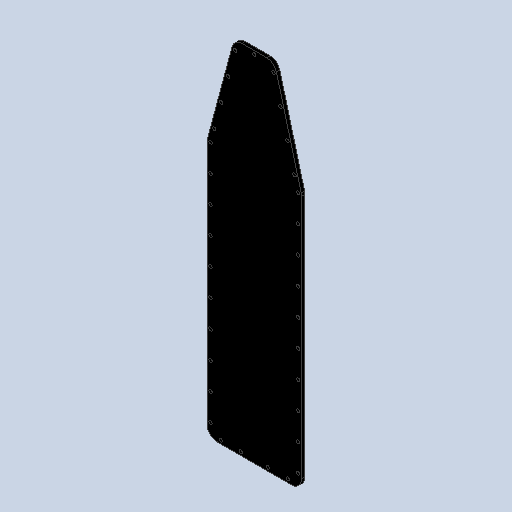
# Autodesk Inventor part: Model Shell - access panel L
Saved by Autodesk Inventor 2023 (Build 270158000, 158)
## iProperties
Created: 2022-12-13
Part Number: Model Shell - access panel L
Material: ABS Plastic
Document SubType Name: Modeling
Designer: Tanzu
Density: 1.06 g/cm^3
Appearance: Aluminum - Polished
Mass: 375.26 g
Surface Area: 1823.85 cm^2
Volume: 354.019 cm^3
Author: Tanzu
Autodesk Inventor part; units mm, degrees
ref_plane "YZ Plane" through (0, 0, 0) normal (1, 0, 0) x (0, 1, 0)
ref_plane "XZ Plane" through (0, 0, 0) normal (0, 1, 0) x (-1, 0, 0)
ref_plane "XY Plane" through (0, 0, 0) normal (0, 0, 1) x (1, 0, 0)
sketch "Sketch2" plane through (0, 0, 0) normal (0, 0, 1) x (1, 0, 0)
  line L0 (-90, 0) -> (90, 0) construction
  line L1 (90, 0) -> (90, 900) construction
  line L2 (90, 900) -> (-90, 900) construction
  line L3 (-90, 900) -> (-90, 0) construction
  line L4 (-90, 250) -> (90, 250) construction
  line L5 (0, 900) -> (90, 564.1154)
  line L6 (0, 900) -> (-90, 564.1154)
  line L7 (0, 900) -> (0, 250) construction
  line L8 (-132.5, 0) -> (132.5, 0) construction
  line L9 (-90, 564.1154) -> (-90, 0)
  line L10 (90, 564.1154) -> (90, 0)
  line L11 (90, 0) -> (-90, 0)
  line L12 (-85, 563.4572) -> (0, 880.6815)
  line L13 (0, 880.6815) -> (85, 563.4572)
  line L14 (85, 563.4572) -> (85, 5)
  line L15 (85, 5) -> (-85, 5)
  line L16 (-85, 5) -> (-85, 563.4572)
  point P0 (0, 0)
  point P1 (0, 0)
  dimension "d4" = 180
  dimension "d5" = 900
  dimension "d6" = 250
  dimension "d7" = 15
  dimension "d8" = 15
  dimension "d9" = 265
  dimension "d10" = 5
  constraints: 34 end point, 4 midpoint, 4 point on line, 3 collinear, 2 horizontal, 2 parallel, 2 perpendicular, 1 coincident, 4 other
  measures "d4" distance of L0.start L0.end
  measures "d5" distance of L0.end L1.end
  measures "d6" distance between parallel lines of L0 L4
  measures "d7" angle of L7 L5
  measures "d8" angle of L6 L7
  measures "d9" distance of L8.start L8.end
  measures "d10" distance between parallel lines of L6 L12
extrude "Extrusion2" add sketch "Sketch2" along normal mid plane 180 contours L5 L10 L11 L9 L6 | L12 L13 L14 L15 L16
sketch "Sketch3" plane through (0, 0, 0) normal (0, 0, 1) x (1, 0, 0)
  line L0 (-132.5, 0) -> (132.5, 0)
  line L1 (-90, 0) -> (90, 0) projected
  line L2 (0, 0) -> (0, 600)
  line L3 (0, 600) -> (-132.5, 0)
  line L4 (0, 601.0824) -> (0, 600)
  line L5 (0, 577.3585) -> (-127.5, 0)
  line L6 (0, 577.3585) -> (0, 601.0824)
  point P0 (0, 0)
  dimension "d13" = 265
  dimension "d14" = 600
  dimension "d17" = 5
  constraints: 12 end point, 3 point on line, 2 midpoint, 2 vertical, 1 collinear, 1 horizontal, 1 parallel
  measures "d13" distance of L0.start L0.end
  measures "d14" distance of L2.start L2.end
  measures "d17" distance of L0.start L5.end
revolve "Revolution1" add sketch "Sketch3" angle 360 about axis through (0, 0, 0) along (0, 1, 0)
revolve "Revolution2" cut sketch "Sketch3" angle 360 about axis through (0, 0, 0) along (0, 1, 0) contours L5 L2 L0
extrude "Extrusion3" cut sketch "Sketch2" along normal mid plane 170 contours L12 L13 L14 L15 L16
sketch "Sketch5" plane through (0, 0, 0) normal (0, -1, 0) x (1, 0, 0)
  circle A0 centre (0, 0) radius 127.5 projected
  circle A1 centre (0, 0) radius 132.5 projected
extrude "Extrusion4" add sketch "Sketch5" along normal blind 100
fillet "Fillet1" radius 10 5 edges at (0, 192.4528, -90) (90, 192.4528, 0) (0, 192.4528, 90) (-90, 152.2344, -40.9581) (-90, 152.2344, 40.9581)
fillet "Fillet2" radius 30 2 edges at (0, 0, 132.5) (0, 0, -132.5)
sketch "Sketch6" plane through (90, 564.1154, 90) normal (1, 0, 0) x (0, 0, -1)
  line L0 (180, 0) -> (180, -526.9621) projected
  line L1 (180, 0) -> (0, 0) projected
  line L2 (0, -526.9621) -> (0, 0) projected
  line L3 (27.5, -275) -> (152.5, -275)
  line L4 (152.5, -275) -> (152.5, -75)
  line L5 (152.5, -75) -> (27.5, -75)
  line L6 (27.5, -75) -> (27.5, -275)
  point P0 (90, -564.1154)
  point P1 (90, 0)
  point P2 (90, -75)
  dimension "d25" = 75
  dimension "d26" = 200
  dimension "d27" = 125
  constraints: 8 end point, 2 midpoint, 2 parallel, 1 horizontal, 1 horizontal alignment, 1 perpendicular, 1 vertical alignment
  measures "d25" distance between parallel lines of L1 L5
  measures "d26" distance of L5.end L3.start
  measures "d27" distance of L3.start L3.end
extrude "Extrusion5" cut sketch "Sketch6" against normal up to next
sketch "Sketch7" plane through (85, 33.0197, 85) normal (-1, 0, 0) x (0, 0, 1)
  line L0 (-22.5, 256.0957) -> (-22.5, 456.0957) projected
  line L1 (-147.5, 256.0957) -> (-22.5, 256.0957) projected
  line L2 (-147.5, 456.0957) -> (-147.5, 256.0957) projected
  line L3 (-22.5, 456.0957) -> (-147.5, 456.0957) projected
  line L4 (-32.5, 446.0957) -> (-32.5, 266.0957)
  line L5 (-32.5, 266.0957) -> (-137.5, 266.0957)
  line L6 (-137.5, 266.0957) -> (-137.5, 446.0957)
  line L7 (-137.5, 446.0957) -> (-32.5, 446.0957)
  point P0 (-85, -33.0197)
  dimension "d30" = 10
  constraints: 8 end point, 3 other
  measures "d30" distance between parallel lines of L0 L4
extrude "Extrusion6" add sketch "Sketch7" against normal blind 3
fillet "Fillet3" radius 5 8 edges at (89, 289.1154, 62.5) (86.5, 299.1154, 52.5) (89, 289.1154, -62.5) (86.5, 299.1154, -52.5) (89, 489.1154, 62.5) (86.5, 479.1154, 52.5) (89, 489.1154, -62.5) (86.5, 479.1154, -52.5)
sketch "Sketch8" plane through (0, 0, -90) normal (0, 0, -1) x (-1, 0, 0)
  line L0 (90, 37.1533) -> (90, 564.1154) projected
  line L1 (90, 564.1154) -> (0, 900) projected
  line L2 (0, 900) -> (-90, 564.1154) projected
  line L3 (-90, 564.1154) -> (-90, 37.1533) projected
  line L4 (-90, 564.1154) -> (0, 900) projected
  line L5 (-20.0962, 825) -> (20.0962, 825)
  line L6 (0, 900) -> (90, 564.1154) projected
  point P0 (0, 0)
  point P1 (20.0962, 825)
  dimension "d34" = 75
  constraints: 2 end point, 2 point on line, 1 horizontal, 1 horizontal alignment
  measures "d34" distance from line of L1.end L5
extrude "Extrusion7" cut sketch "Sketch8" against normal through all
sketch "Sketch9" plane through (0, 0, -90) normal (0, 0, -1) x (-1, 0, 0)
  line L0 (20.0962, 825) -> (-20.0962, 825) projected
  line L1 (-20.0962, 825) -> (-90, 564.1154) projected
  line L2 (-90, 564.1154) -> (-90, 37.1533) projected
  line L3 (90, 37.1533) -> (90, 564.1154) projected
  line L4 (90, 564.1154) -> (20.0962, 825) projected
  line L5 (-55, 164.1154) -> (55, 164.1154)
  line L6 (70, 179.1154) -> (70, 542.1406)
  line L7 (70, 544.1154) -> (-70, 544.1154) construction
  line L8 (-70, 542.1406) -> (-70, 179.1154)
  line L9 (-69.4889, 546.0229) -> (-32.7866, 682.9977)
  line L10 (-18.2977, 694.1154) -> (18.2977, 694.1154)
  line L11 (-90, 37.1533) -> (-90, 564.1154) projected
  line L12 (32.7866, 682.9977) -> (69.4889, 546.0229)
  line L13 (-20.0962, 825) -> (-90, 564.1154) projected
  line L14 (90, 564.1154) -> (20.0962, 825) projected
  arc A0 (-70, 179.1154) -> (-55, 164.1154) centre (-55, 179.1154) ccw
  arc A1 (55, 164.1154) -> (70, 179.1154) centre (55, 179.1154) ccw
  arc A2 (-18.2977, 694.1154) -> (-32.7866, 682.9977) centre (-18.2977, 679.1154) ccw
  arc A3 (32.7866, 682.9977) -> (18.2977, 694.1154) centre (18.2977, 679.1154) ccw
  arc A4 (-69.4889, 546.0229) -> (-70, 542.1406) centre (-55, 542.1406) ccw
  arc A5 (70, 542.1406) -> (69.4889, 546.0229) centre (55, 542.1406) ccw
  line L15 (70, 542.1406) -> (70, 544.1154) construction
  line L16 (70, 544.1154) -> (69.4889, 546.0229) construction
  line L17 (-70, 542.1406) -> (-70, 544.1154) construction
  line L18 (-69.4889, 546.0229) -> (-70, 544.1154) construction
  line L19 (-65, 179.1154) -> (-65, 542.1406) construction
  arc A6 (-64.6593, 544.7288) -> (-65, 542.1406) centre (-55, 542.1406) ccw construction
  line L20 (-64.6593, 544.7288) -> (-27.957, 681.7036) construction
  arc A7 (-18.2977, 689.1154) -> (-27.957, 681.7036) centre (-18.2977, 679.1154) ccw construction
  line L21 (-18.2977, 689.1154) -> (18.2977, 689.1154) construction
  arc A8 (27.957, 681.7036) -> (18.2977, 689.1154) centre (18.2977, 679.1154) ccw construction
  line L22 (27.957, 681.7036) -> (64.6593, 544.7288) construction
  arc A9 (65, 542.1406) -> (64.6593, 544.7288) centre (55, 542.1406) ccw construction
  line L23 (65, 542.1406) -> (65, 179.1154) construction
  arc A10 (55, 169.1154) -> (65, 179.1154) centre (55, 179.1154) ccw construction
  line L24 (55, 169.1154) -> (-55, 169.1154) construction
  arc A11 (-65, 179.1154) -> (-55, 169.1154) centre (-55, 179.1154) ccw construction
  line L25 (-60, 542.1406) -> (-60, 179.1154)
  arc A12 (-60, 179.1154) -> (-55, 174.1154) centre (-55, 179.1154) ccw
  line L26 (-55, 174.1154) -> (55, 174.1154)
  arc A13 (55, 174.1154) -> (60, 179.1154) centre (55, 179.1154) ccw
  line L27 (60, 179.1154) -> (60, 542.1406)
  arc A14 (60, 542.1406) -> (59.8296, 543.4347) centre (55, 542.1406) ccw
  line L28 (59.8296, 543.4347) -> (23.1273, 680.4095)
  arc A15 (23.1273, 680.4095) -> (18.2977, 684.1154) centre (18.2977, 679.1154) ccw
  line L29 (18.2977, 684.1154) -> (-18.2977, 684.1154)
  arc A16 (-18.2977, 684.1154) -> (-23.1273, 680.4095) centre (-18.2977, 679.1154) ccw
  line L30 (-23.1273, 680.4095) -> (-59.8296, 543.4347)
  arc A17 (-59.8296, 543.4347) -> (-60, 542.1406) centre (-55, 542.1406) ccw
  circle A18 centre (-65, 184.1154) radius 2.5
  circle A19 centre (65, 184.1154) radius 2.5
  circle A20 centre (-65, 224.1154) radius 2.5
  circle A21 centre (65, 224.1154) radius 2.5
  circle A22 centre (-65, 264.1154) radius 2.5
  circle A23 centre (65, 264.1154) radius 2.5
  circle A24 centre (-65, 304.1154) radius 2.5
  circle A25 centre (65, 304.1154) radius 2.5
  circle A26 centre (-65, 344.1154) radius 2.5
  circle A27 centre (65, 344.1154) radius 2.5
  circle A28 centre (-65, 384.1154) radius 2.5
  circle A29 centre (65, 384.1154) radius 2.5
  circle A30 centre (-50, 169.1154) radius 2.5
  circle A31 centre (-20, 169.1154) radius 2.5
  circle A32 centre (-59.4646, 564.1154) radius 2.5
  circle A33 centre (-49.1119, 602.7525) radius 2.5
  circle A34 centre (-38.7591, 641.3895) radius 2.5
  circle A35 centre (-28.4063, 680.0265) radius 2.5
  circle A36 centre (0, 689.1154) radius 2.5
  line L31 (0, 164.1154) -> (0, 174.1154) construction
  circle A37 centre (50, 169.1154) radius 2.5
  circle A38 centre (20, 169.1154) radius 2.5
  circle A39 centre (59.4646, 564.1154) radius 2.5
  circle A40 centre (49.1119, 602.7525) radius 2.5
  circle A41 centre (38.7591, 641.3895) radius 2.5
  circle A42 centre (28.4063, 680.0265) radius 2.5
  line L32 (-249.5323, -205.2434) -> (226.5579, -205.2434)
  line L33 (226.5579, -205.2434) -> (226.5579, 884.6963)
  line L34 (226.5579, 884.6963) -> (-249.5323, 884.6963)
  line L35 (-249.5323, 884.6963) -> (-249.5323, -205.2434)
  circle A43 centre (-65, 424.1154) radius 2.5
  circle A44 centre (65, 424.1154) radius 2.5
  circle A45 centre (-65, 464.1154) radius 2.5
  circle A46 centre (65, 464.1154) radius 2.5
  circle A47 centre (-65, 504.1154) radius 2.5
  circle A48 centre (65, 504.1154) radius 2.5
  circle A49 centre (-65, 544.1154) radius 2.5
  circle A50 centre (65, 544.1154) radius 2.5
  point P0 (0, 0)
  dimension "d37" = 20
  dimension "d38" = 20
  dimension "d39" = 20
  dimension "d41" = 150
  dimension "d42" = 15
  dimension "d43" = 15
  dimension "d44" = 15
  dimension "d45" = 15
  dimension "d46" = 15
  dimension "d47" = 15
  dimension "d48" = 380
  dimension "d49" = 5
  dimension "d50" = 5
  dimension "d51" = 5
  dimension "d52" = 5
  dimension "d53" = 10
  dimension "d59" = 40
  dimension "d63" = 5
  dimension "d64" = 15
  dimension "d70" = 30
  dimension "d72" = 5
  dimension "d79" = 40
  dimension "d81" = 5
  dimension "d190" = 20
  constraints: 56 end point, 51 centre point, 36 point on circle, 14 tangent, 8 parallel, 6 symmetric about line, 5 horizontal, 5 perpendicular, 5 vertical, 4 point on line, 3 midpoint, 2 horizontal alignment, 1 collinear, 73 other
  measures "d37" distance between parallel lines of L2 L8
  measures "d38" distance between parallel lines of L3 L6
  measures "d39" distance from line of L1.end L7
  measures "d41" distance between parallel lines of L7 L10
  measures "d42" radius of A1
  measures "d43" radius of A0
  measures "d44" radius of A4
  measures "d45" radius of A5
  measures "d46" radius of A2
  measures "d47" radius of A3
  measures "d48" distance between parallel lines of L7 L5
  measures "d49" distance between parallel lines of L8 L19
  measures "d50" distance between parallel lines of L25 L19
  measures "d51" diameter of A18
  measures "d52" diameter of A19
  measures "d53" distance from line of A18.centre L26
  measures "d59" distance of A18.centre A20.centre
  measures "d63" diameter of A30
  measures "d64" distance from line of L19 A30.centre
  measures "d70" distance of A30.centre A31.centre
  measures "d72" diameter of A32
  measures "d79" distance of A32.centre A33.centre
  measures "d81" diameter of A36
  measures "d190" vertical distance of A49.centre A32.centre
extrude "Extrusion10" cut sketch "Sketch9" along normal through all both and the other way through all contours A0 L8 A4 L9 A2 L10 A3 L12 A5 L6 A1 L5 | A17 L30 A16 L29 A15 L28 A14 L27 A13 L26 A12 L25 | A18 | A19 | A20 | A21 | A22 | A23 | A24 | A25 | A26 | A27 | A28 | A29 | A30 | A31 | A32 | A33 | A34 | A35 | A36 | A37 | A38 | A39 | A40 | A41 | A42 | L35 L34 L33 L32 | A43 | A44 | A45 | A46 | A47 | A48 | A49 | A50
extrude "Extrusion11" add sketch "Sketch9" against normal blind 5 contours A0 L8 A4 L9 A2 L10 A3 L12 A5 L6 A1 L5 | A17 L30 A16 L29 A15 L28 A14 L27 A13 L26 A12 L25
chamfer "Chamfer3" distance 2 angle 45 33 edges at (67.5, 184.1154, -90) (67.5, 224.1154, -90) (67.5, 264.1154, -90) (67.5, 304.1154, -90) (67.5, 344.1154, -90) (52.5, 169.1154, -90) (22.5, 169.1154, -90) (-17.5, 169.1154, -90) (-47.5, 169.1154, -90) (-62.5, 184.1154, -90) (-62.5, 224.1154, -90) (-62.5, 264.1154, -90) (-62.5, 304.1154, -90) (-62.5, 344.1154, -90) (-62.5, 384.1154, -90) (-56.9646, 564.1154, -90) (-46.6119, 602.7525, -90) (-36.2591, 641.3895, -90) (-25.9063, 680.0265, -90) (2.5, 689.1154, -90) (30.9063, 680.0265, -90) (41.2591, 641.3895, -90) (51.6119, 602.7525, -90) (61.9646, 564.1154, -90) (67.5, 384.1154, -90) (67.5, 424.1154, -90) (67.5, 464.1154, -90) (67.5, 504.1154, -90) (-62.5, 504.1154, -90) (-62.5, 464.1154, -90) (-62.5, 424.1154, -90) (-62.5, 544.1154, -90) (67.5, 544.1154, -90)
ref_plane "Work Plane1" through (-55, 214.1154, -90) normal (0, -1, 0) x (1, 0, 0)
sketch "Sketch13" plane through (-55, 214.1154, -90) normal (0, -1, 0) x (1, 0, 0)
  line L0 (125, 0) -> (110, 0) projected
  line L1 (125, 0) -> (125, 5) projected
  line L2 (110, 5) -> (125, 5) projected
  line L3 (110, 0) -> (110, 5) projected
  line L4 (125.5, 6) -> (116, 6)
  line L5 (115.5, -1) -> (125.5, -1)
  line L6 (126, -0.5) -> (126, 5.5)
  arc A0 (126, 5.5) -> (125.5, 6) centre (125.5, 5.5) ccw
  arc A1 (125.5, -1) -> (126, -0.5) centre (125.5, -0.5) ccw
  line L7 (116, 6) -> (116, 5)
  line L8 (124.4889, 5) -> (87.7866, 5) projected
  line L9 (115.5, -1) -> (115.5, 0)
  line L10 (125, 0) -> (126, 0)
  point P0 (55, 90)
  point P1 (126, 6)
  dimension "d182" = 1
  dimension "d183" = 1
  dimension "d184" = 1
  dimension "d185" = 10
  dimension "d186" = 0.5
  dimension "d187" = 10
  constraints: 12 end point, 5 point on line, 4 point on circle, 4 tangent, 3 perpendicular, 2 centre point, 1 equal radius, 1 horizontal, 1 parallel
  measures "d182" distance between parallel lines of L4 L2
  measures "d183" distance between parallel lines of L6 L1
  measures "d184" distance between parallel lines of L0 L5
  measures "d185" distance of point (126, 6) L4.end
  measures "d186" radius of A0
  measures "d187" distance of L5.start L5.end
sketch3d "3D Sketch1"
  line L0 (70, 179.1154, -90) -> (70, 542.1406, -90)
  arc A0 (70, 542.1406, -90) -> (69.4889, 546.0229, -90) centre (55, 542.1406, -90) ccw
  line L1 (69.4889, 546.0229, -90) -> (32.7866, 682.9977, -90)
  arc A1 (32.7866, 682.9977, -90) -> (18.2977, 694.1154, -90) centre (18.2977, 679.1154, -90) ccw
  line L2 (18.2977, 694.1154, -90) -> (-18.2977, 694.1154, -90)
  arc A2 (-18.2977, 694.1154, -90) -> (-32.7866, 682.9977, -90) centre (-18.2977, 679.1154, -90) ccw
  line L3 (-32.7866, 682.9977, -90) -> (-69.4889, 546.0229, -90)
  arc A3 (-69.4889, 546.0229, -90) -> (-70, 542.1406, -90) centre (-55, 542.1406, -90) ccw
  line L4 (-70, 542.1406, -90) -> (-70, 179.1154, -90)
  arc A4 (-70, 179.1154, -90) -> (-55, 164.1154, -90) centre (-55, 179.1154, -90) ccw
  line L5 (-55, 164.1154, -90) -> (55, 164.1154, -90)
  arc A5 (55, 164.1154, -90) -> (70, 179.1154, -90) centre (55, 179.1154, -90) ccw
sweep "Sweep1" add profiles "Sketch13" path "3D Sketch1" separate body contours L1 L2 L7 L4 A0 L6 L10
body "Solid2"
body "Solid3"
